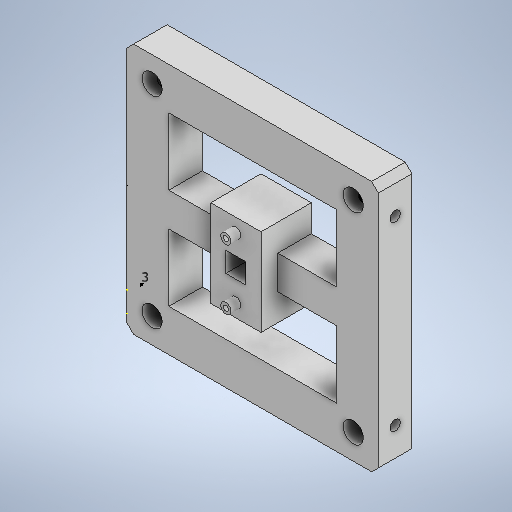
# Autodesk Inventor part: camera_60mm
Saved by Autodesk Inventor 2025.1 (Build 291241000, 241)
## iProperties
Created: 2024-11-22
Part Number: camera_60mm
Material: Ogólny
Document SubType Name: Modeling
Designer: PC
Density: 1 g/cm^3
Appearance: Domyślna
Author: PC
Autodesk Inventor part; units mm, degrees
ref_plane "YZ Plane" through (0, 0, 0) normal (1, 0, 0) x (0, 1, 0)
ref_plane "XZ Plane" through (0, 0, 0) normal (0, 1, 0) x (-1, 0, 0)
ref_plane "XY Plane" through (0, 0, 0) normal (0, 0, 1) x (1, 0, 0)
sketch "Szkic1" plane through (0, 0, 0) normal (0, 0, 1) x (1, 0, 0)
  line L0 (-24.2993, 7.2735) -> (25.7007, 7.2735) construction
  circle A0 centre (60, 60) radius 3
  circle A1 centre (0, 60) radius 3
  line L1 (40, 45) -> (20, 45) construction
  line L2 (20, 45) -> (20, 15) construction
  line L3 (20, 15) -> (40, 15) construction
  line L4 (40, 15) -> (40, 45) construction
  line L5 (40, 45) -> (20, 15) construction
  line L6 (20, 45) -> (40, 15) construction
  line L7 (30, 45) -> (30, 15) construction
  circle A2 centre (30, 39) radius 0.75
  circle A3 centre (30, 21) radius 0.75
  circle A4 centre (30, 39) radius 1.5
  circle A5 centre (30, 21) radius 1.5
  line L8 (22.5, 17) -> (37.5, 17)
  line L9 (33, 33) -> (27, 33)
  line L10 (27, 33) -> (27, 27)
  line L11 (27, 27) -> (33, 27)
  line L12 (33, 27) -> (33, 33)
  line L13 (33, 33) -> (27, 27) construction
  line L14 (27, 33) -> (33, 27) construction
  line L15 (30, 39) -> (30, 21) construction
  line L16 (0, 60) -> (60, 60) construction
  line L17 (60, 60) -> (60, 0) construction
  line L18 (60, 0) -> (0, 0) construction
  line L19 (0, 0) -> (0, 60) construction
  circle A6 centre (0, 0) radius 3
  circle A7 centre (60, 0) radius 3
  line L20 (22.5, 43) -> (37.5, 43)
  line L21 (-7.5, 67.5) -> (67.5, 67.5)
  line L22 (67.5, 67.5) -> (67.5, -7.5)
  line L23 (67.5, -7.5) -> (-7.5, -7.5)
  line L24 (-7.5, -7.5) -> (-7.5, 67.5)
  line L25 (-7.5, 67.5) -> (67.5, -7.5) construction
  line L26 (67.5, 67.5) -> (-7.5, -7.5) construction
  line L27 (5, 55) -> (55, 55)
  line L28 (55, 5) -> (5, 5)
  line L29 (5, 35) -> (22.5, 35)
  line L30 (22.5, 25) -> (5, 25)
  line L31 (37.5, 35) -> (55, 35)
  line L32 (55, 25) -> (37.5, 25)
  line L33 (22.5, 17) -> (22.5, 25)
  line L34 (22.5, 35) -> (22.5, 43)
  line L35 (37.5, 43) -> (37.5, 35)
  line L36 (37.5, 25) -> (37.5, 17)
  line L37 (5, 5) -> (5, 25)
  line L38 (5, 35) -> (5, 55)
  line L39 (55, 55) -> (55, 35)
  line L40 (55, 25) -> (55, 5)
  line L41 (5, 55) -> (5, 5) construction
  line L42 (55, 5) -> (55, 55) construction
  line L43 (22.5, 35) -> (22.5, 25)
  line L44 (37.5, 25) -> (37.5, 35)
  point P0 (30, 30)
  point P1 (37.6222, 60)
  point P2 (33, 30)
  point P3 (60, 30)
  point P4 (30, 27)
  point P5 (30, 0)
  point P6 (30, 30)
  point P7 (5, 30)
  point P8 (-7.5, 30)
  point P9 (30, 5)
  point P10 (30, -7.5)
  point P11 (30, 43)
  dimension "d3" = 20
  dimension "d4" = 30
  dimension "d5" = 1.5
  dimension "d6" = 18
  dimension "d7" = 3
  dimension "d8" = 3
  dimension "d9" = 6
  dimension "d10" = 6
  dimension "d11" = 15
  dimension "d14" = 60
  dimension "d15" = 60
  dimension "d16" = 6
  dimension "d19" = 75
  dimension "d20" = 75
  dimension "d21" = 50
  dimension "d22" = 10
  dimension "d23" = 10
  dimension "d24" = 10
  constraints: 90 end point, 18 midpoint, 16 parallel, 12 perpendicular, 8 centre point, 8 horizontal, 8 point on line, 6 coincident, 6 collinear, 4 equal radius, 4 horizontal alignment, 3 vertical alignment, 1 vertical
  measures "d3" distance of L3.end L2.end
  measures "d4" distance of L2.end L1.end
  measures "d5" diameter of A2
  measures "d6" distance of A3.centre A2.centre
  measures "d7" diameter of A4
  measures "d8" diameter of A5
  measures "d9" distance of L11.end L9.start
  measures "d10" distance of L10.end L11.end
  measures "d11" distance of L8.start L8.end
  measures "d14" distance of L17.end L18.end
  measures "d15" distance of L16.end L17.end
  measures "d16" diameter of A1
  measures "d19" distance of L22.end L23.end
  measures "d20" distance of L21.end L22.end
  measures "d21" distance of L27.start L27.end
  measures "d22" distance between parallel lines of L9 L20
  measures "d23" distance between parallel lines of L8 L11
  measures "d24" distance between parallel lines of L30 L29
extrude "Wyciągnięcie proste1" add sketch "Szkic1" along normal blind 15 contours L33 L43 L34 L20 L35 L44 L36 L8
extrude "Wyciągnięcie proste2" add sketch "Szkic1" along normal blind 18 contours A4 | A5
extrude "Wyciągnięcie proste3" add sketch "Szkic1" along normal blind 10 contours L21 L22 L23 L24
chamfer "Faza1" distance 2 angle 45 4 edges at (67.5, 67.5, 5) (67.5, -7.5, 5) (-7.5, -7.5, 5) (-7.5, 67.5, 5)
sketch "Szkic2" plane through (-7.5, -5.5, 0) normal (-1, 0, 0) x (0, 0, 1)
  line L0 (10, 8.5) -> (0, 8.5) projected
  line L1 (10, 2.5) -> (0, 2.5) projected
  circle A0 centre (5, 8.5) radius 1.5
  line L2 (0, 71) -> (0, 0) construction
  line L3 (0, 35.5) -> (10, 35.5) construction
  circle A1 centre (5, 62.5) radius 1.5
  point P0 (0, 5.5)
  point P1 (5, 2.5)
  dimension "d34" = 3
  constraints: 4 midpoint, 2 centre point, 2 end point, 1 horizontal, 1 symmetric about line, 1 vertical alignment, 1 other
  measures "d34" diameter of A0
extrude "Wyciągnięcie proste4" cut sketch "Szkic2" against normal blind 15
extrude "Wyciągnięcie proste5" cut sketch "Szkic2" against normal up to surface (12.5 mm away) from surface at -62.5
